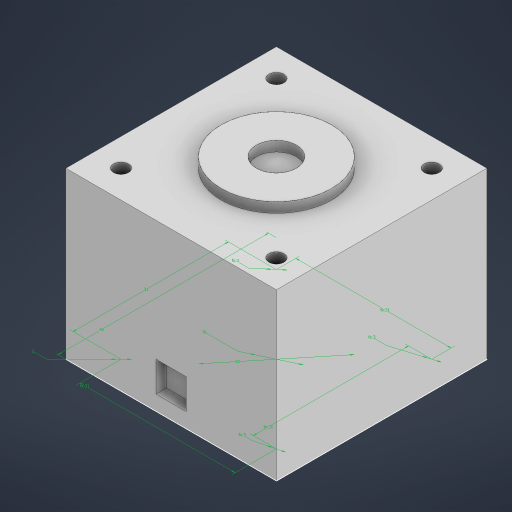
# Autodesk Inventor part: NEMA17 Stepper Motor
Saved by Autodesk Inventor 2024.2 (Build 282272000, 272)
## iProperties
Created: 2024-10-02
Part Number: NEMA17 Stepper Motor
Material: Generic
Document SubType Name: Modeling
Designer: jerem
Density: 1 g/cm^3
Appearance: Default
Author: jerem
Autodesk Inventor part; units mm, degrees
ref_plane "YZ Plane" through (0, 0, 0) normal (1, 0, 0) x (0, 1, 0)
ref_plane "XZ Plane" through (0, 0, 0) normal (0, 1, 0) x (-1, 0, 0)
ref_plane "XY Plane" through (0, 0, 0) normal (0, 0, 1) x (1, 0, 0)
sketch "Sketch1" plane through (0, 0, 0) normal (0, 1, 0) x (-1, 0, 0)
  line L0 (-21, -21) -> (21, -21)
  line L1 (21, -21) -> (21, 21)
  line L2 (21, 21) -> (-21, 21)
  line L3 (-21, 21) -> (-21, -21)
  line L4 (-21, -21) -> (21, 21) construction
  line L5 (21, -21) -> (-21, 21) construction
  circle A0 centre (15.5, 15.5) radius 1.5
  circle A1 centre (15.5, -15.5) radius 1.5
  circle A2 centre (-15.5, -15.5) radius 1.5
  circle A3 centre (-15.5, 15.5) radius 1.5
  circle A4 centre (0, 0) radius 11
  circle A5 centre (0, 0) radius 4
  dimension "d0" = 42
  dimension "d1" = 31
  dimension "d2" = 31
  dimension "d3" = 31
  dimension "d4" = 31
  dimension "d5" = 3
  dimension "d6" = 3
  dimension "d7" = 3
  dimension "d8" = 3
  dimension "d11" = 22
  dimension "d14" = 8
  constraints: 12 end point, 6 centre point, 4 point on line, 2 coincident, 2 midpoint, 2 parallel, 2 perpendicular, 1 horizontal
  measures "d0" distance of L0.end L1.end
  measures "d1" distance of A1.centre A0.centre
  measures "d2" distance of A2.centre A1.centre
  measures "d3" distance of A3.centre A2.centre
  measures "d4" distance of A0.centre A3.centre
  measures "d5" diameter of A0
  measures "d6" diameter of A1
  measures "d7" diameter of A2
  measures "d8" diameter of A3
  measures "d11" diameter of A4
  measures "d14" diameter of A5
extrude "Extrusion1" add sketch "Sketch1" along normal blind 33 contours L3 L2 L1 L0 | A4 | A5
extrude "Extrusion2" add sketch "Sketch1" along normal blind 2 from surface at 33 contours A4 | A5
extrude "Extrusion3" cut sketch "Sketch1" against normal blind 2 from surface at 35 contours A5
sketch "Sketch2" plane through (-21, 0, 21) normal (0, 0, 1) x (1, 0, 0)
  line L0 (24, 9) -> (18, 9)
  line L1 (18, 9) -> (18, 3)
  line L2 (18, 3) -> (24, 3)
  line L3 (24, 3) -> (24, 9)
  line L4 (24, 9) -> (18, 3) construction
  line L5 (18, 9) -> (24, 3) construction
  line L6 (0, 0) -> (42, 0) projected
  line L7 (42, 0) -> (42, 33) projected
  line L8 (0, 0) -> (0, 33) projected
  point P0 (21, 0)
  point P1 (21, 6)
  point P2 (21, 0)
  dimension "d17" = 6
  dimension "d18" = 6
  dimension "d19" = 3
  dimension "d20" = 18
  dimension "d21" = 18
  constraints: 12 end point, 3 midpoint, 2 parallel, 1 horizontal, 1 perpendicular
  measures "d17" distance of L2.end L1.end
  measures "d18" distance of L1.end L0.end
  measures "d19" distance from line of point (21, 0) L2
  measures "d20" distance between parallel lines of L7 L3
  measures "d21" distance between parallel lines of L8 L1
extrude "Extrusion4" cut sketch "Sketch2" against normal blind 2
equation "\"d2\" = d1"
equation "\"d3\" = d1"
equation "\"d4\" = d1"
equation "\"d6\" = d5"
equation "\"d7\" = d5"
equation "\"d8\" = d5"
body "Solid1"
